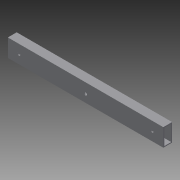
# Autodesk Inventor part: Drive base
Saved by Autodesk Inventor 2015 (Build 190159000, 159)
## iProperties
Created: 2015-10-07
Part Number: Drive base
Material: Generic
Document SubType Name: Modeling
Designer: alhohbein
Density: 1 g/cm^3
Appearance: Default
Author: alhohbein
Autodesk Inventor part; units mm, degrees
ref_plane "YZ Plane" through (0, 0, 0) normal (1, 0, 0) x (0, 1, 0)
ref_plane "XZ Plane" through (0, 0, 0) normal (0, 1, 0) x (-1, 0, 0)
ref_plane "XY Plane" through (0, 0, 0) normal (0, 0, 1) x (1, 0, 0)
sketch "Sketch1" plane through (0, 0, 0) normal (0, 0, 1) x (1, 0, 0)
  line L0 (222.25, 25.4) -> (-222.25, 25.4)
  line L1 (-222.25, 25.4) -> (-222.25, -25.4)
  line L2 (-222.25, -25.4) -> (222.25, -25.4)
  line L3 (222.25, -25.4) -> (222.25, 25.4)
  line L4 (222.25, 25.4) -> (-222.25, -25.4) construction
  line L5 (-222.25, 25.4) -> (222.25, -25.4) construction
  point P0 (0, 0)
  dimension "d0" = 444.5
  dimension "d1" = 50.8
  constraints: 12 end point, 2 midpoint, 2 parallel, 1 horizontal, 1 perpendicular
  measures "d0" distance of L2.end L1.end
  measures "d1" distance of L1.end L0.end
extrude "Extrusion1" add sketch "Sketch1" along normal blind 25.4
sketch "Sketch2" plane through (0, 0, 25.4) normal (0, 0, 1) x (1, 0, 0)
  point P0 (0, -3.175)
  point P1 (0, -3.175)
  point P2 (-190.5, 0)
  point P3 (190.5, 0)
  point P4 (0, 0)
  dimension "d4" = 3.175
  dimension "d5" = 190.5
  dimension "d6" = 190.5
  dimension "d7" = 3.175
  constraints: 1 coincident, 1 horizontal alignment, 1 vertical alignment
  measures "d4" vertical distance of point (0, -3.175) point (190.5, 0)
  measures "d5" horizontal distance of point (190.5, 0) point (0, -3.175)
  measures "d6" horizontal distance of point (-190.5, 0) point (0, -3.175)
  measures "d7" distance of point (0, 0) point (0, -3.175)
shell "Shell1" thickness 2.54 removed faces 2 at (222.25, -8.4667, 8.4667) at (-222.25, 8.4667, 16.9333)
hole "Hole1" at (0, -3.175, 25.4) at (-190.5, 0, 25.4) at (190.5, 0, 25.4) direction (0, 0, -1) diameter 8.1026 end through all
equation "\"d6\" = d5"
body "Solid1"
